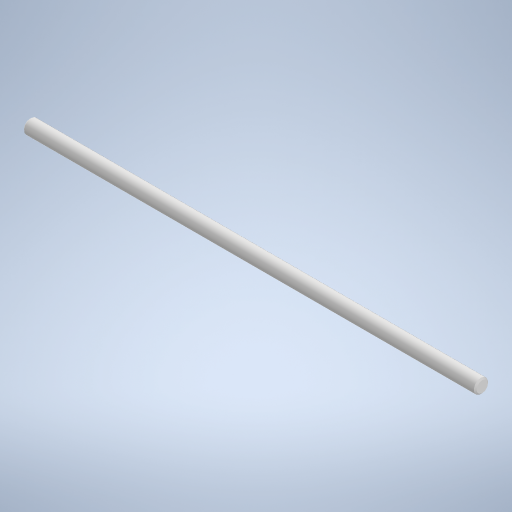
# Autodesk Inventor part: Staaf
Saved by Autodesk Inventor 2023 (Build 270158000, 158)
## iProperties
Created: 2022-12-05
Part Number: Staaf
Material: Generic
Document SubType Name: Modeling
Designer: Ayoub
Density: 1 g/cm^3
Appearance: Default
Author: Ayoub
Autodesk Inventor part; units mm, degrees
ref_plane "YZ Plane" through (0, 0, 0) normal (1, 0, 0) x (0, 1, 0)
ref_plane "XZ Plane" through (0, 0, 0) normal (0, 1, 0) x (-1, 0, 0)
ref_plane "XY Plane" through (0, 0, 0) normal (0, 0, 1) x (1, 0, 0)
sketch "Sketch2" plane through (0, 0, 0) normal (1, 0, 0) x (0, 1, 0)
  circle A0 centre (0, 0) radius 5
  dimension "d6" = 10
  constraints: 1 centre point, 1 coincident
  measures "d6" diameter of A0
extrude "Extrusion2" add sketch "Sketch2" along normal blind 320
chamfer "Chamfer2" distance 1 angle 45 2 edges at (0, -5, 0) (320, -5, 0)
body "Solid2"
